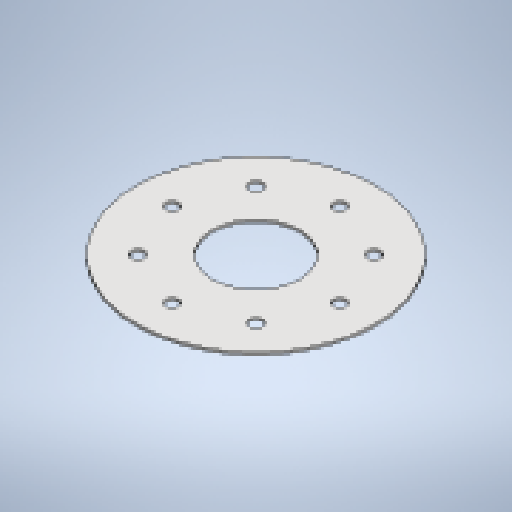
# Autodesk Inventor part: TKS 3109 top DS main flange
Saved by Autodesk Inventor 2025.3 (Build 293356030, 356C)
## iProperties
Created: 2024-12-09
Part Number: TKS 3109 top DS main flange
Material: Stainless Steel
Document SubType Name: Sheet Metal
Designer: user
Mass: 3269.02 g
Surface Area: 1007.63 cm^2
Volume: 408.627 cm^3
Density: 8 g/cm^3
Flat Pattern Width: 32 cm
Flat Pattern Length: 32 cm
Flat Pattern Area: 1024 cm^2
Sheet Metal Rule: AISI304 3mm Die 32
Sheet Metal Width: 320,000 mm
Sheet Metal Length: 320,000 mm
Sheet Metal Area: 102400,000 mm^2
Appearance: Default
Author: user
Autodesk Inventor part; units mm, degrees
ref_plane "YZ Plane" through (0, 0, 0) normal (1, 0, 0) x (0, 1, 0)
ref_plane "XZ Plane" through (0, 0, 0) normal (0, 1, 0) x (-1, 0, 0)
ref_plane "XY Plane" through (0, 0, 0) normal (0, 0, 1) x (1, 0, 0)
sketch "Sketch1" plane through (0, 0, 0) normal (0, 0, 1) x (1, 0, 0)
  circle A0 centre (0, 0) radius 72.5
  circle A1 centre (0, 0) radius 160
  dimension "d22" = 145
  dimension "d23" = 320
  measures "d22" diameter of A0
  measures "d23" diameter of A1
extrude "Plate1" add sketch "Sketch1" along normal blind 4
sketch "Sketch5" plane through (0, 0, 4) normal (0, 0, 1) x (1, 0, 0)
  circle A0 centre (0, 140) radius 11
  circle A1 centre (0, 0) radius 140 construction
  circle A2 centre (0, 0) radius 190 construction
  circle A3 centre (0, 190) radius 6.5
  dimension "d25" = 280
  dimension "d32" = 380
  dimension "d24" = 22
  dimension "d31" = 13
  constraints: 4 vertical alignment, 2 centre point, 2 coincident, 4 other
  measures "d24" diameter of A0
  measures "d31" diameter of A3
extrude "Cut1" cut sketch "Sketch5" against normal blind 4 contours A0
pattern_circular "Circular Pattern1" count 8 over 360 about axis through (0, 0, 0) along (0, 0, 1) of "Cut1"
equation "\"d26\" = Thickness"
equation "\"d2\" = Thickness"
equation "\"BendReliefWidth\" = Thickness"
equation "\"BendReliefDepth\" = 0.5 * Thickness"
equation "\"CornerReliefSize\" = 4 * Thickness"
equation "\"MinimumRemnant\" = 2 * Thickness"
equation "\"TransitionRadius\" = BendRadius"
equation "\"JacobiRadiusSize\" = BendRadius"
equation "\"GapSize\" = Thickness"
equation "\"Thickness\" = 4"
equation "\"BendRadius\" = 5"
body "Solid1"
